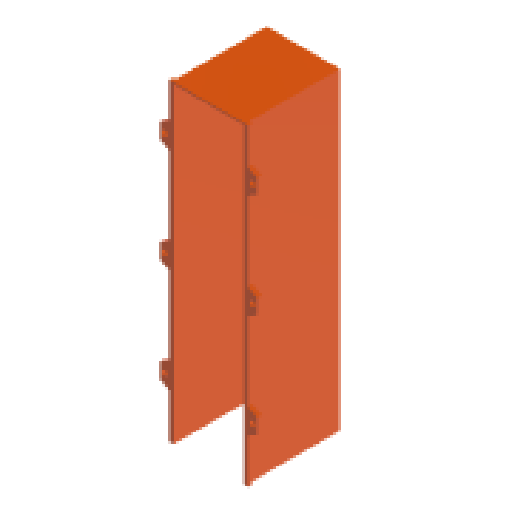
# Autodesk Inventor part: Drag Chain Cover
Saved by Autodesk Inventor 2023.2 (Build 272271000, 271)
## iProperties
Created: 2023-02-24
Part Number: Drag Chain Cover
Material: ABS Plastic
Document SubType Name: Modeling
Designer: remop
Density: 1.06 g/cm^3
Appearance: Smooth - Light Orange
Author: remop
Autodesk Inventor part; units mm, degrees
ref_plane "YZ Plane" through (0, 0, 0) normal (1, 0, 0) x (0, 1, 0)
ref_plane "XZ Plane" through (0, 0, 0) normal (0, 1, 0) x (-1, 0, 0)
ref_plane "XY Plane" through (0, 0, 0) normal (0, 0, 1) x (1, 0, 0)
sketch "Sketch1" plane through (0, 0, 0) normal (0, 0, 1) x (1, 0, 0)
  line L0 (-23.512, 105) -> (23.512, 105)
  line L1 (23.512, 105) -> (23.512, -105)
  line L2 (23.512, -105) -> (-23.512, -105)
  line L3 (-23.512, -105) -> (-23.512, 105)
  line L4 (-23.512, 105) -> (23.512, -105) construction
  line L5 (23.512, 105) -> (-23.512, -105) construction
  line L6 (-24.712, 106.2) -> (24.712, 106.2)
  line L7 (24.712, 106.2) -> (24.712, -106.2)
  line L8 (24.712, -106.2) -> (-24.712, -106.2)
  line L9 (-24.712, -106.2) -> (-24.712, 106.2)
  line L10 (-24.712, 106.2) -> (24.712, -106.2) construction
  line L11 (24.712, 106.2) -> (-24.712, -106.2) construction
  line L12 (23.512, -105) -> (24.712, -105)
  line L13 (-23.512, -105) -> (-24.712, -105)
  point P0 (0, 0)
  dimension "d0" = 47.024
  dimension "d1" = 210
  dimension "d2" = 1.2
  dimension "d3" = 1.2
  constraints: 28 end point, 4 midpoint, 4 parallel, 3 horizontal, 3 perpendicular, 2 point on line
  measures "d0" distance of L1.end L2.end
  measures "d1" distance of L0.end L1.end
  measures "d2" distance between parallel lines of L7 L1
  measures "d3" distance between parallel lines of L0 L6
extrude "Extrusion1" add sketch "Sketch1" along normal blind 64 contours L3 L13 L9 L6 L7 L12 L1 L0
sketch "Sketch2" plane through (0, 0, 64) normal (0, 0, 1) x (1, 0, 0)
  line L0 (23.512, -105) -> (24.712, -105) projected
  line L1 (24.712, -105) -> (24.712, 106.2) projected
  line L2 (24.712, 106.2) -> (-24.712, 106.2) projected
  line L3 (-24.712, 106.2) -> (-24.712, -105) projected
  line L4 (-24.712, -105) -> (-23.512, -105) projected
  line L5 (-23.512, -105) -> (-23.512, 105) projected
  line L6 (-23.512, 105) -> (23.512, 105) projected
  line L7 (23.512, 105) -> (23.512, -105) projected
  circle A0 centre (-29.712, -66.5359) radius 1.85
  line L8 (-24.712, -105) -> (-26.712, -105)
  line L9 (-26.712, -105) -> (-26.712, -75)
  line L10 (-32.712, -61.5359) -> (-32.712, -71.5359)
  line L11 (-32.712, -71.5359) -> (-26.712, -75)
  line L12 (-32.712, -61.5359) -> (-26.712, -58.0718)
  line L13 (-26.712, -75) -> (-26.712, -58.0718) construction
  line L14 (-32.712, 8.4641) -> (-26.712, 11.9282)
  line L15 (-32.712, 8.4641) -> (-32.712, -1.5359)
  line L16 (-32.712, -1.5359) -> (-26.712, -5)
  line L17 (-26.712, -5) -> (-26.712, 11.9282) construction
  circle A1 centre (-29.712, 3.4641) radius 1.85
  line L18 (-32.712, 78.4641) -> (-26.712, 81.9282)
  line L19 (-32.712, 78.4641) -> (-32.712, 68.4641)
  line L20 (-32.712, 68.4641) -> (-26.712, 65)
  line L21 (-26.712, 65) -> (-26.712, 81.9282) construction
  circle A2 centre (-29.712, 73.4641) radius 1.85
  line L22 (-26.712, -58.0718) -> (-26.712, -5)
  line L23 (-26.712, 11.9282) -> (-26.712, 65)
  line L24 (-26.712, 81.9282) -> (-26.712, 106.2)
  line L25 (-26.712, 106.2) -> (-24.712, 106.2)
  point P0 (0, 0)
  point P1 (-32.712, -66.5359)
  point P2 (-32.712, 3.4641)
  point P3 (-32.712, 73.4641)
  dimension "d6" = 3.7
  dimension "d7" = 5
  dimension "d8" = 3
  dimension "d9" = 10
  dimension "d10" = 60
  dimension "d11" = 60
  dimension "d12" = 30
  dimension "d13" = 2
  dimension "d16" = 70
  constraints: 36 end point, 4 vertical, 3 centre point, 2 perpendicular, 1 collinear, 1 horizontal, 1 horizontal alignment, 1 midpoint, 1 point on line, 22 other
  measures "d6" diameter of A0
  measures "d7" distance from line of L3 A0.centre
  measures "d8" distance from line of A0.centre L10
  measures "d9" distance of L10.start L10.end
  measures "d10" angle of L10 L11
  measures "d11" angle of L10 L12
  measures "d12" distance of L9.end L8.end
  measures "d13" distance of L3.end L8.end
  measures "d16" distance of L10.start L14.start
extrude "Extrusion2" add sketch "Sketch2" against normal blind 3 contours L3 L8 L9 L11 L10 L12 L22 L16 L15 L14 L23 L20 L19 L18 L24 L25
mirror "Mirror1" about plane through (0, 0, 0) normal (1, 0, 0) of "Extrusion2"
equation "\"d3\" = d2"
equation "\"d11\" = d10"
body "Solid1"
